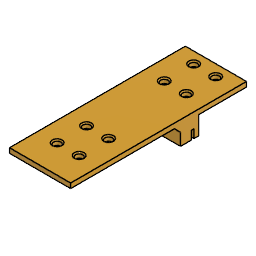
Plataforma_Péndulo (Autodesk Fusion 360 design; units mm, degrees)
Autodesk Fusion 360 part; units mm, degrees
sketch "Boceto1" plane through (0, 0, 0) normal (0, 0, 1) x (1, 0, 0)
  line L0 (-12.3094, 26.9942) -> (17.6906, 26.9942)
  line L1 (17.6906, 26.9942) -> (17.6906, -7.0058)
  line L2 (17.6906, -7.0058) -> (-12.3094, -7.0058)
  line L3 (-12.3094, -7.0058) -> (-12.3094, 26.9942)
  line L4 (-12.3094, 9.9942) -> (17.6906, 9.9942) construction
  line L5 (2.6906, 9.9942) -> (2.6906, -2.0058) construction
  line L6 (2.6906, -2.0058) -> (-6.3094, -2.0058) construction
  circle A0 centre (-6.3094, -2.0058) radius 2
  circle A1 centre (11.6906, -2.0058) radius 2
  circle A2 centre (-6.3094, 21.9942) radius 2
  circle A3 centre (11.6906, 21.9942) radius 2
  line L7 (-12.3094, -60.5058) -> (17.6906, -60.5058)
  line L8 (17.6906, -60.5058) -> (17.6906, -94.5058)
  line L9 (17.6906, -94.5058) -> (-12.3094, -94.5058)
  line L10 (-12.3094, -94.5058) -> (-12.3094, -60.5058)
  line L11 (-12.3094, -77.5058) -> (17.6906, -77.5058) construction
  line L12 (2.6906, -77.5058) -> (2.6906, -89.5058) construction
  line L13 (2.6906, -89.5058) -> (-6.3094, -89.5058) construction
  circle A4 centre (-6.3094, -89.5058) radius 2
  line L14 (2.6906, 9.9942) -> (2.6906, -77.5058) construction
  line L15 (27.6906, -98.7558) -> (-22.3094, -98.7558)
  line L16 (-22.3094, -98.7558) -> (-22.3094, 31.2442)
  line L17 (-22.3094, 31.2442) -> (27.6906, 31.2442)
  line L18 (27.6906, 31.2442) -> (27.6906, -98.7558)
  line L19 (27.6906, -98.7558) -> (-22.3094, 31.2442) construction
  line L20 (-22.3094, -98.7558) -> (27.6906, 31.2442) construction
  circle A5 centre (11.6906, -89.5058) radius 2
  circle A6 centre (-6.3094, -65.5058) radius 2
  circle A7 centre (11.6906, -65.5058) radius 2
  circle A8 centre (-6.3094, -2.0058) radius 3
  circle A9 centre (11.6906, -2.0058) radius 3
  circle A10 centre (-6.3094, 21.9942) radius 3
  circle A11 centre (11.6906, 21.9942) radius 3
  line L21 (2.6906, -33.7558) -> (27.6906, -33.7558) construction
  circle A12 centre (11.6906, -65.5058) radius 3
  circle A13 centre (11.6906, -89.5058) radius 3
  circle A14 centre (-6.3094, -89.5058) radius 3
  circle A15 centre (-6.3094, -65.5058) radius 3
  line L22 (-22.3094, -94.5058) -> (27.6906, -94.5058)
  line L23 (27.6906, -94.5058) -> (27.6906, -112.5058)
  line L24 (27.6906, -112.5058) -> (-22.3094, -112.5058)
  line L25 (-22.3094, -112.5058) -> (-22.3094, -94.5058)
  point P0 (-12.3094, 26.9942)
  point P1 (-12.3094, 26.9942)
  point P2 (-27.1477, -6.5825)
  point P3 (-27.1477, -6.5825)
  point P4 (2.6906, -33.7558)
  dimension "d25" = 30
  dimension "d26" = 34
  dimension "d28" = 12
  dimension "d29" = 9
  dimension "d30" = 4
  dimension "d32" = 30
  dimension "d33" = 34
  dimension "d34" = 12
  dimension "d35" = 9
  dimension "d36" = 4
  dimension "d37" = 53.5
  dimension "d38" = 130
  dimension "d39" = 50
  dimension "d42" = 6
  dimension "d70" = 18
  constraint coincident P1 P0
  constraint horizontal L0
  constraint vertical L1
  constraint horizontal L2
  constraint vertical L3
  constraint midpoint L3 L4.start
  constraint midpoint L1 L4.end
  constraint midpoint L4 L5.start
  constraint perpendicular L4 L5
  constraint perpendicular L5 L6
  constraint coincident L6.end A0.centre
  constraint symmetric L5 A0 A1
  constraint symmetric L4 A0 A2
  constraint symmetric L4 A1 A3
  constraint horizontal L7
  constraint vertical L8
  constraint horizontal L9
  constraint vertical L10
  constraint midpoint L10 L11.start
  constraint midpoint L8 L11.end
  constraint midpoint L11 L12.start
  constraint perpendicular L11 L12
  constraint perpendicular L12 L13
  constraint coincident L13.end A4.centre
  constraint perpendicular L11 L14
  constraint horizontal L15
  constraint perpendicular L15 L16
  constraint parallel L15 L17
  constraint parallel L16 L18
  constraint coincident L19 P4
  constraint coincident L20 P4
  constraint midpoint L14 P4
  constraint symmetric L12 A4 A5
  constraint symmetric L11 A4 A6
  constraint symmetric L11 A5 A7
  constraint concentric A0 A8
  constraint symmetric L14 A8 A9
  constraint symmetric L4 A8 A10
  constraint symmetric L4 A9 A11
  constraint coincident P4 L21.start
  constraint midpoint L18 L21.end
  constraint symmetric A8 L21 A15
  constraint symmetric A9 L21 A12
  constraint symmetric A10 L21 A14
  constraint symmetric A11 L21 A13
  constraint horizontal L22
  constraint vertical L23
  constraint horizontal L24
  constraint vertical L25
  constraint coincident L16 L22.start
  measures "d25" distance of P1 L0.end
  measures "d26" distance of L0 L2
  measures "d28" distance of L5.start L5.end
  measures "d29" distance of L5.end L6.end
  measures "d30" diameter of A0
  measures "d32" distance of L7.start L7.end
  measures "d33" distance of L7.start L9.end
  measures "d34" distance of L12.start L12.end
  measures "d35" distance of L12.end L13.end
  measures "d36" diameter of A4
  measures "d37" distance of L2 L7
  measures "d38" distance of L15.start L17.end
  measures "d39" distance of L16.end L17.end
  measures "d42" diameter of A8
  measures "d70" distance of L22.start L24.end
extrude "Extrude2" add sketch "Boceto1" along normal blind 4 contours L0 L1 L2 L3 | L7 L8 L10 L16 L17 L18 L22 | L7 L8 L9 L10 L22 | L9 L15 L16 L18 L22 L23 L25 | L15 L23 L24 L25
sketch "Sketch3" plane through (0, 0, 4) normal (0, 0, 1) x (-1, 0, 0)
  line L0 (-27.6906, -31.2442) -> (22.3094, -31.2442)
  line L1 (22.3094, -31.2442) -> (22.3094, 112.5058)
  line L2 (-27.6906, 112.5058) -> (-27.6906, -31.2442)
  line L3 (-11.6906, 2.0058) -> (-11.6906, 5.0058)
  line L4 (-27.6906, -31.2442) -> (-27.6906, 7.7558)
  line L5 (36.9053, 13.2102) -> (36.9053, 38.2102)
  line L6 (40.9053, 37.6992) -> (40.9053, 38.2102)
  line L7 (40.9053, 35.7102) -> (40.9053, 15.7102)
  line L8 (40.9053, 15.7102) -> (42.9053, 15.7102)
  line L9 (48.9053, 38.2102) -> (48.9053, 13.2102)
  line L10 (42.9053, 15.7102) -> (42.9053, 35.7102)
  line L11 (48.9053, 13.2102) -> (36.9053, 38.2102) construction
  line L12 (40.9053, 37.6992) -> (40.9053, 35.7102)
  line L13 (36.9053, 38.2102) -> (48.9053, 38.2102)
  line L14 (40.9053, 15.7102) -> (40.9053, 13.2102)
  line L15 (42.9053, 15.7102) -> (42.9053, 13.2102)
  line L16 (48.9053, 13.2102) -> (36.9053, 13.2102)
  line L17 (42.9053, 35.7102) -> (42.8232, 35.7102)
  spline S0 degree 5 poles (42.9053, 35.7102) (43.1525, 35.6842) (43.6233, 35.6158) (44.2591, 35.4635) (44.9637, 35.1596) (45.5917, 34.6019) (45.9513, 33.8551) (46.0336, 32.913) (45.8513, 31.7846) (45.4286, 30.487) (44.7911, 29.0381) (44.1263, 27.7699) (43.5468, 26.7619) (43.125, 26.0649) (42.9053, 25.7102) knots 0 0 0 0 0 0 0.1 0.2 0.3 0.4 0.5 0.6 0.7 0.8 0.9 1 1 1 1 1 1
  line L18 (36.9053, 13.2102) -> (48.9053, 38.2102) construction
  spline S1 degree 3 poles (43.1142, 37.6992) (44.1976, 37.5855) (45.2054, 37.3255) (46.1041, 36.7178) (46.7989, 36.2481) (47.395, 35.5241) (47.6958, 34.7009) (48.0554, 33.7167) (48.0255, 32.6966) (47.8334, 31.7152) (47.5191, 30.1091) (46.7761, 28.4673) (45.7624, 26.6285) (45.4119, 25.9925) (45.0261, 25.3359) (44.6056, 24.657) knots 0 0 0 0 0.211284 0.211284 0.211284 0.37461 0.37461 0.37461 0.569894 0.569894 0.569894 0.88947 0.88947 0.88947 1 1 1 1
  arc A0 (44.6056, 24.657) -> (42.9053, 21.0364) centre (47.6105, 21.0364) ccw
  line L19 (43.1142, 37.6992) -> (43.1142, 38.2102)
  line L20 (-27.6906, 7.7558) -> (22.3094, 7.7558)
  line L21 (22.3094, 7.7558) -> (22.3094, 22.7558)
  line L22 (22.3094, 22.7558) -> (-27.6906, 22.7558)
  line L23 (-27.6906, 22.7558) -> (-27.6906, 7.7558)
  line L24 (22.3094, 7.7558) -> (22.3094, 11.7558)
  line L25 (22.3094, 11.7558) -> (-2.6906, 11.7558)
  line L26 (-2.6906, 11.7558) -> (-2.6906, 13.7558)
  line L27 (22.3094, 13.7558) -> (22.3094, 11.7558)
  line L28 (-27.6906, 7.7558) -> (-27.6906, 11.7558)
  line L29 (-27.6906, 11.7558) -> (-2.6906, 11.7558)
  line L30 (-2.6906, 11.7558) -> (-2.6906, 13.7558)
  line L31 (-2.6906, 13.7558) -> (-27.6906, 13.7558)
  line L32 (-27.6906, 13.7558) -> (-27.6906, 11.7558)
  spline S2 degree 5 poles (42.9053, 35.7102) (43.1525, 35.6842) (43.6233, 35.6158) (44.2591, 35.4635) (44.9637, 35.1596) (45.5917, 34.6019) (45.9513, 33.8551) (46.0336, 32.913) (45.8513, 31.7846) (45.4286, 30.487) (44.7911, 29.0381) (44.1263, 27.7699) (43.5468, 26.7619) (43.125, 26.0649) (42.9053, 25.7102) knots 0 0 0 0 0 0 0.1 0.2 0.3 0.4 0.5 0.6 0.7 0.8 0.9 1 1 1 1 1 1
  spline S3 degree 5 poles (9.9506, 13.7558) (9.7826, 14.0404) (9.4386, 14.58) (8.8989, 15.3006) (8.1354, 16.0878) (7.1251, 16.801) (6.0795, 17.2616) (5.0167, 17.4838) (3.9473, 17.4752) (2.8696, 17.2384) (1.7734, 16.7695) (0.8709, 16.2009) (0.1741, 15.6605) (-0.3001, 15.2486) (-0.5395, 15.0297) knots 0 0 0 0 0 0 0.1 0.2 0.3 0.4 0.5 0.6 0.7 0.8 0.9 1 1 1 1 1 1
  spline S4 degree 3 poles (12.5339, 15.2812) (11.2696, 17.4223) (9.5599, 19.0305) (7.5918, 19.8385) (5.8063, 20.5716) (3.8266, 20.6251) (2.0306, 20.063) (0.3684, 19.5428) (-1.1234, 18.5602) (-2.5634, 17.2442) knots 0 0 0 0 0.364047 0.364047 0.364047 0.694319 0.694319 0.694319 1 1 1 1
  line L33 (-2.5634, 17.2442) -> (-2.6906, 13.7558)
  arc A1 (12.5339, 15.2812) -> (16.2316, 13.7558) centre (16.2316, 19.0004) ccw
  line L34 (-2.6906, 13.7558) -> (9.9506, 13.7558)
  line L35 (16.2316, 13.7558) -> (22.3094, 13.7558)
  line L36 (-2.6906, -9.9942) -> (-2.6906, 77.5058)
  spline S5 degree 5 poles (-15.3319, 13.7558) (-15.1639, 14.0404) (-14.8199, 14.58) (-14.2802, 15.3006) (-13.5167, 16.0878) (-12.5064, 16.801) (-11.4608, 17.2616) (-10.398, 17.4838) (-9.3286, 17.4752) (-8.2509, 17.2384) (-7.1547, 16.7695) (-6.2522, 16.2009) (-5.5554, 15.6605) (-5.0812, 15.2486) (-4.8417, 15.0297) knots 0 0 0 0 0 0 0.1 0.2 0.3 0.4 0.5 0.6 0.7 0.8 0.9 1 1 1 1 1 1
  line L37 (10.6601, 12.5543) -> (9.2411, 14.9573)
  line L38 (0.4984, 15.9782) -> (-1.5775, 14.0812)
  line L39 (-16.0414, 12.5543) -> (-14.6224, 14.9573)
  line L40 (-5.8796, 15.9782) -> (-3.8038, 14.0812)
  spline S6 degree 3 poles (-17.9152, 15.2812) (-16.6509, 17.4223) (-14.9412, 19.0305) (-12.9731, 19.8385) (-11.1876, 20.5716) (-9.2079, 20.6251) (-7.4119, 20.063) (-5.7497, 19.5428) (-4.2579, 18.5602) (-2.8179, 17.2442) knots 0 0 0 0 0.364047 0.364047 0.364047 0.694319 0.694319 0.694319 1 1 1 1
  arc A2 (-21.6129, 13.7558) -> (-17.9152, 15.2812) centre (-21.6129, 19.0004) ccw
  line L41 (-2.8179, 17.2442) -> (-2.6906, 13.7558)
  line L42 (22.3094, 112.5058) -> (-27.6906, 112.5058)
  circle A3 centre (-11.6906, 2.0058) radius 3
  circle A4 centre (6.3094, 2.0058) radius 3
  circle A5 centre (-11.6906, 65.5058) radius 3
  circle A6 centre (6.3094, -21.9942) radius 3
  circle A7 centre (-11.6906, 89.5058) radius 3
  circle A8 centre (-11.6906, -21.9942) radius 3
  circle A9 centre (6.3094, 65.5058) radius 3
  circle A10 centre (6.3094, 89.5058) radius 3
  line L43 (-2.5634, 17.2442) -> (-2.8179, 17.2442)
  arc A11 (-0.5395, 15.0297) -> (-0.9099, 13.7558) centre (0.3202, 14.0889) ccw
  line L44 (-0.9099, 13.7558) -> (-3.8038, 14.0812)
  arc A12 (-4.8417, 13.7558) -> (-4.8417, 15.0297) centre (-5.4239, 14.3928) ccw
  line L45 (-4.8417, 13.7558) -> (1.2796, 10.3603)
  point P0 (42.9053, 25.7102)
  point P1 (40.9053, 15.7102)
  point P2 (45.9053, 33.7102)
  point P3 (45.9053, 33.7102)
  point P4 (4.9873, 17.4288)
  point P5 (-10.3686, 17.4288)
  dimension "d46" = 39
  dimension "d5" = -2
  dimension "d48" = 2
  dimension "d49" = 20
  dimension "d50" = 12
  dimension "d51" = 25
  dimension "d52" = 4
  dimension "d53" = 50
  dimension "d54" = 15
  dimension "d55" = 4
  dimension "d56" = 25
  dimension "d57" = 4
  dimension "d58" = 2
  dimension "d59" = 2.5
  dimension "d60" = 3
  dimension "d61" = 4
  dimension "d76" = 7
  constraint vertical L3
  constraint coincident L0.start L2.end
  constraint perpendicular L0 L4
  constraint vertical L10
  constraint vertical L7
  constraint coincident P1 L7.end
  constraint midpoint P0 L10
  constraint horizontal L16
  constraint perpendicular L5 L16
  constraint parallel L13 L16
  constraint parallel L5 L9
  constraint coincident P0 L11
  constraint coincident P0 L18
  constraint coincident P0 S0.end
  constraint vertical L12
  constraint horizontal L17
  constraint midpoint L15.end L16
  constraint coincident L14.end L16
  constraint perpendicular L14 L16
  constraint perpendicular L8 L10
  constraint coincident L19.end L13
  constraint perpendicular L13 L19
  constraint coincident L6.end L13
  constraint perpendicular L6 L13
  constraint tangent L10 A0
  constraint coincident A0.end L10
  constraint horizontal L20
  constraint vertical L21
  constraint horizontal L22
  constraint vertical L23
  constraint perpendicular L20 L24
  constraint horizontal L25
  constraint vertical L26
  constraint horizontal L34
  constraint vertical L27
  constraint perpendicular L20 L28
  constraint horizontal L29
  constraint vertical L30
  constraint horizontal L31
  constraint vertical L32
  constraint tangent A1 L34
  constraint coincident A1.end L34
  constraint collinear L34 L35
  constraint midpoint S3.start L37
  constraint midpoint S3.end L38
  constraint symmetric L26.end L36 L30.end
  constraint symmetric S3.end L36 S5.end
  constraint symmetric S3.start L36 S5.start
  constraint symmetric P4 L36 P5
  constraint symmetric S4.start L36 S6.start
  constraint symmetric S4.end L36 S6.end
  constraint symmetric S4 L36 S6
  constraint symmetric A1.end L36 A2.start
  constraint symmetric A1 L36 A2
  constraint symmetric L36 L37.start L39.start
  constraint symmetric L36 L37.end L39.end
  constraint symmetric L36 L38.start L40.start
  constraint symmetric L36 L38.end L40.end
  constraint coincident L34 A11.end
  constraint tangent S3 A11
  constraint coincident L40.end L44.end
  constraint coincident L31 A12.start
  constraint tangent S5 A12
  measures "d46" distance of L0.start L4.end
  measures "d48" distance of P1 L8.end
  measures "d49" distance of L7.start P1
  measures "d50" distance of L5.end L9.start
  measures "d51" distance of L5.end L5.start
  measures "d52" distance of A0.end S1.end
  measures "d53" distance of L4.end L20.end
  measures "d54" distance of L4.end L22.end
  measures "d55" distance of L20.end L24.end
  measures "d56" distance of L24.end L25.end
  measures "d57" distance of L4.end L28.end
  measures "d58" distance of L29 L31
  measures "d59" distance of L26.end S3.end
  measures "d61" distance of S4.start A1.end
  measures "d76" distance of A12.start L45.end
extrude "Extrude4" add sketch "Sketch3" along normal blind 15 contours L2 L20 L23 L28 L29 L36 | L1 L20 L21 L24 L25 L36 | S3 L34 A11 | L2 L22 L23 L31 L36 S6 A2 L43 | L1 L21 L22 S4 A1 L35 L36 L43 | L31 S5 A12
extrude "Extrude5" add sketch "Sketch3" along normal blind 8 contours L2 L23 L26 L29 L30 L31 L32 L36 L45 | L1 L21 L25 L26 L27 L30 S4 L33 A1 L34 L35 L36 L44 L45 | L25 L26 L30 L36 L45 | L31 S5 L40 S6 A2 L41 L44 | L26 L30 L31 L36 L45 | L33 L34 L44 | L31 L40 L41 L44 A12
chamfer "Chaflán5" distance 5 angle 45 1 edges at (2.6906, -22.7558, 4)
fillet "Empalme1" radius 1 8 edges at (-9.1063, -64.421, 0) (-9.1063, -88.421, 0) (8.8937, -88.421, 0) (8.8937, -64.421, 0) (-9.1063, -0.921, 0) (8.8937, -0.921, 0) (8.8937, 23.079, 0) (-9.1063, 23.079, 0)
move_body "Desplazar1" bodies 1 to x (-1, 0, 0) y (0, 1, 0) z (0, 0, -1) at (8.3929, 0, 8)
equation "d37 = 52.5 mm + 1 mm"
